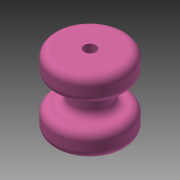
# Autodesk Inventor part: awesome inventor thing
Saved by Autodesk Inventor 2015 (Build 190159000, 159)
## iProperties
Created: 2014-11-30
Part Number: awesome inventor thing
Material: Rock Wool
Document SubType Name: Modeling
Designer: srinis
Density: 0.2 g/cm^3
Appearance: Magenta
Author: srinis
Autodesk Inventor part; units mm, degrees
ref_plane "YZ Plane" through (0, 0, 0) normal (1, 0, 0) x (0, 1, 0)
ref_plane "XZ Plane" through (0, 0, 0) normal (0, 1, 0) x (-1, 0, 0)
ref_plane "XY Plane" through (0, 0, 0) normal (0, 0, 1) x (1, 0, 0)
sketch "Sketch1" plane through (0, 0, 0) normal (0, 1, 0) x (-1, 0, 0)
  circle A0 centre (0, 0) radius 15
  dimension "d0" = 30
  constraints: 1 centre point, 1 coincident
  measures "d0" diameter of A0
extrude "Extrusion1" add sketch "Sketch1" along normal blind 10
sketch "Sketch2" plane through (0, 10, 0) normal (0, 1, 0) x (1, 0, 0)
  circle A0 centre (0, 0) radius 7.5
  dimension "d3" = 15
  constraints: 1 centre point, 1 coincident
  measures "d3" diameter of A0
extrude "Extrusion2" add sketch "Sketch2" along normal blind 10
sketch "Sketch3" plane through (0, 20, 0) normal (0, 1, 0) x (1, 0, 0)
  circle A0 centre (0, 0) radius 15
  dimension "d6" = 30
  constraints: 1 centre point, 1 coincident
  measures "d6" diameter of A0
extrude "Extrusion3" add sketch "Sketch3" along normal blind 10
fillet "Fillet1" radius 3.175 1 edges at (-15, 30, 0)
fillet "Fillet2" radius 3.175 1 edges at (-15, 20, 0)
fillet "Fillet3" radius 3.175 1 edges at (15, 10, 0)
fillet "Fillet4" radius 3.175 1 edges at (15, 0, 0)
fillet "Fillet5" radius 3.175 1 edges at (-7.5, 20, 0)
fillet "Fillet6" radius 3.175 1 edges at (-7.5, 10, 0)
hole "Hole1" at (0, 30, 0) direction (0, -1, 0) diameter 5 end through all
body "Solid1"
